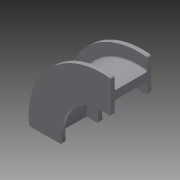
# Autodesk Inventor part: Curved 100mm
Saved by Autodesk Inventor 2015 (Build 190159000, 159)
## iProperties
Created: 2016-12-13
Part Number: Curved 100mm
Material: Generic
Document SubType Name: Modeling
Designer: Rudge-Top
Density: 1 g/cm^3
Appearance: Default
Author: Rudge-Top
Autodesk Inventor part; units mm, degrees
ref_plane "YZ Plane" through (0, 0, 0) normal (1, 0, 0) x (0, 1, 0)
ref_plane "XZ Plane" through (0, 0, 0) normal (0, 1, 0) x (-1, 0, 0)
ref_plane "XY Plane" through (0, 0, 0) normal (0, 0, 1) x (1, 0, 0)
sketch "Sketch1" plane through (0, 0, 0) normal (0, 1, 0) x (-1, 0, 0)
  line L0 (0, 0) -> (141.4214, 0) construction
  line L1 (100, 0) -> (0, 0)
  arc A0 (100.1961, -98.1961) -> (1.8039, 0.1961) centre (10.63, -89.37) ccw
  arc A1 (59.9366, -97.6681) -> (2.3319, -40.0634) centre (10.63, -89.37) ccw
  line L2 (98.2058, -100) -> (61.9088, -100)
  line L3 (0, -1.7942) -> (0, -38.0912)
  arc A2 (98.2058, -100) -> (100.1961, -98.1961) centre (98.2058, -98) ccw
  arc A3 (59.9366, -97.6681) -> (61.9088, -100) centre (61.9088, -98) ccw
  arc A4 (0, -38.0912) -> (2.3319, -40.0634) centre (2, -38.0912) ccw
  arc A5 (1.8039, 0.1961) -> (0, -1.7942) centre (2, -1.7942) ccw
  point P0 (100, -100)
  point P1 (59.4869, -100)
  point P2 (0, -40.5131)
  dimension "d2" = 100
  dimension "d3" = 90
  dimension "d4" = 40
  dimension "d7" = 2
  constraints: 16 point on circle, 8 end point, 8 tangent, 6 centre point, 4 point on line, 3 equal radius, 2 horizontal, 1 vertical
  measures "d2" horizontal distance of point (100, -100) L0.start
  measures "d3" radius of A0
  measures "d4" radial gap between concentric circles of A0 A1
  measures "d7" radius of A2
extrude "Extrusion1" add sketch "Sketch1" along normal blind 5
sketch "Sketch2" plane through (0, 5, 0) normal (0, 1, 0) x (1, 0, 0)
  arc A0 (-98.2058, 100) -> (-100.1961, 98.1961) centre (-98.2058, 98) ccw projected
  arc A1 (-100.1961, 98.1961) -> (-1.8039, -0.1961) centre (-10.63, 89.37) ccw projected
  arc A2 (-1.8039, -0.1961) -> (0, 1.7942) centre (-2, 1.7942) ccw projected
  line L0 (0, 1.7942) -> (0, 38.0912) projected
  arc A3 (0, 38.0912) -> (-2.3319, 40.0634) centre (-2, 38.0912) ccw projected
  arc A4 (-59.9366, 97.6681) -> (-2.3319, 40.0634) centre (-10.63, 89.37) ccw projected
  arc A5 (-59.9366, 97.6681) -> (-61.9088, 100) centre (-61.9088, 98) ccw projected
  line L1 (-61.9088, 100) -> (-98.2058, 100) projected
  arc A6 (-84.8728, 100) -> (0, 15.1272) centre (-10.63, 89.37) ccw
  arc A7 (-74.7549, 100) -> (0, 25.2451) centre (-10.63, 89.37) ccw
  line L2 (0, 15.1272) -> (0, 25.2451)
  line L3 (-84.8728, 100) -> (-74.7549, 100)
  point P0 (0, 0)
  dimension "d10" = 15
  constraints: 4 end point, 4 point on circle, 4 point on line, 2 centre point, 1 collinear, 1 perpendicular
  measures "d10" radial gap between concentric circles of A1 A6
extrude "Extrusion2" add sketch "Sketch2" along normal blind 40 contours L1 A7 L0 A6
fillet "Fillet1" radius 2 2 edges at (-63.663, 5, -36.337) (-56.5919, 5, -43.4081)
sketch "Sketch3" plane through (0, 45, 0) normal (0, 1, 0) x (1, 0, 0)
  arc A0 (-86.8927, 100) -> (0, 13.1073) centre (-10.63, 89.37) ccw projected
  line L0 (-86.8927, 100) -> (-98.2058, 100) projected
  arc A1 (-98.2058, 100) -> (-100.1961, 98.1961) centre (-98.2058, 98) ccw projected
  arc A2 (-100.1961, 98.1961) -> (-1.8039, -0.1961) centre (-10.63, 89.37) ccw projected
  arc A3 (-1.8039, -0.1961) -> (0, 1.7942) centre (-2, 1.7942) ccw projected
  line L1 (0, 1.7942) -> (0, 13.1073) projected
  arc A4 (-72.7267, 100) -> (0, 27.2733) centre (-10.63, 89.37) ccw projected
  line L2 (0, 27.2733) -> (0, 38.0912) projected
  arc A5 (0, 38.0912) -> (-2.3319, 40.0634) centre (-2, 38.0912) ccw projected
  arc A6 (-59.9366, 97.6681) -> (-2.3319, 40.0634) centre (-10.63, 89.37) ccw projected
  arc A7 (-59.9366, 97.6681) -> (-61.9088, 100) centre (-61.9088, 98) ccw projected
  line L3 (-61.9088, 100) -> (-72.7267, 100) projected
  arc A8 (-84.8728, 100) -> (0, 15.1272) centre (-10.63, 89.37) ccw projected
  line L4 (0, 15.1272) -> (0, 25.2451) projected
  arc A9 (-74.7549, 100) -> (0, 25.2451) centre (-10.63, 89.37) ccw projected
  line L5 (-74.7549, 100) -> (-84.8728, 100) projected
  arc A10 (-74.7549, 100) -> (0, 25.2451) centre (-10.63, 89.37) ccw projected
  arc A11 (-86.8927, 100) -> (0, 13.1073) centre (-10.63, 89.37) ccw projected
  line L6 (0, 27.2733) -> (0, 25.2451)
  line L7 (0, 15.1272) -> (0, 13.1073)
  line L8 (-72.7267, 100) -> (-74.7549, 100)
  line L9 (-74.7549, 100) -> (-84.8728, 100)
  line L10 (-86.8927, 100) -> (-84.8728, 100)
  point P0 (0, 0)
  constraints: 10 end point, 2 collinear, 2 horizontal, 1 vertical
extrude "Extrusion3" add sketch "Sketch3" along normal blind 5
fillet "Fillet2" radius 2 2 edges at (-56.5919, 45, -43.4081) (-63.663, 45, -36.337)
body "Solid1"
